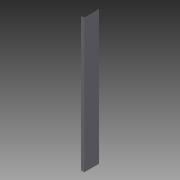
# Autodesk Inventor part: 2014 Sidings
Saved by Autodesk Inventor 2014 (Build 180170000, 170)
## iProperties
Created: 2014-01-17
Part Number: 2014 Sidings
Material: Generic
Document SubType Name: Sheet Metal
Designer: NilesStanton
Density: 1 g/cm^3
Sheet Metal Rule: Default
Appearance: Default
Author: NilesStanton
Autodesk Inventor part; units mm, degrees
ref_plane "YZ Plane" through (0, 0, 0) normal (1, 0, 0) x (0, 1, 0)
ref_plane "XZ Plane" through (0, 0, 0) normal (0, 1, 0) x (-1, 0, 0)
ref_plane "XY Plane" through (0, 0, 0) normal (0, 0, 1) x (1, 0, 0)
sketch "Sketch1" plane through (0, 0, 0) normal (0, 1, 0) x (-1, 0, 0)
  line L0 (0, 0) -> (0, 88.9)
  line L1 (0, 88.9) -> (19.05, 88.9)
  line L2 (19.05, 88.9) -> (19.05, 88.265)
  line L3 (19.05, 88.265) -> (0.635, 88.265)
  line L4 (0.635, 88.265) -> (0.635, 0.635)
  line L5 (0, 0) -> (6.35, 0)
  line L6 (6.35, 0) -> (6.35, 0.635)
  line L7 (6.35, 0.635) -> (0.635, 0.635)
  dimension "d0" = 88.9
  dimension "d1" = 19.05
  dimension "d2" = 0.635
  dimension "d4" = 0.635
  dimension "d7" = 6.35
  constraints: 16 end point, 5 parallel, 3 perpendicular, 1 vertical
  measures "d0" distance of L0.start L0.end
  measures "d1" distance of L0.end L1.end
  measures "d2" distance of L1.end L2.end
  measures "d4" distance between parallel lines of L4 L0
  measures "d7" distance of L0.start L5.end
extrude "Extrusion1" add sketch "Sketch1" along normal blind 812.8
sketch "Sketch2" plane through (-19.05, 0, 88.9) normal (0, 0, 1) x (1, 0, 0)
  line L0 (19.05, 0) -> (0, 0) projected
  line L1 (19.05, 0) -> (19.05, 812.8) projected
  line L2 (9.525, 0) -> (9.525, 12.7)
  line L3 (0, 0) -> (0, 812.8) projected
  line L4 (9.525, 12.7) -> (9.525, 27.5524) construction
  dimension "d8" = 12.7
  constraints: 4 end point, 2 parallel, 1 midpoint
  measures "d8" distance of L2.start L2.end
hole "Hole1" at (-9.525, 12.7, 88.9) direction (0, 0, -1) diameter 2.54 end through all
pattern_linear "Rectangular Pattern1" count 32 spacing 25.4 along (0, 1, 0) of "Hole1"
equation "\"d14\" = Thickness"
equation "\"BendRadius\" = Thickness"
equation "\"BendReliefWidth\" = Thickness"
equation "\"BendReliefDepth\" = 0.5 * Thickness"
equation "\"CornerReliefSize\" = 4 * Thickness"
equation "\"MinimumRemnant\" = 2 * Thickness"
equation "\"TransitionRadius\" = BendRadius"
equation "\"JacobiRadiusSize\" = BendRadius"
equation "\"GapSize\" = Thickness"
equation "\"Thickness\" = 3.048"
body "Solid1"
